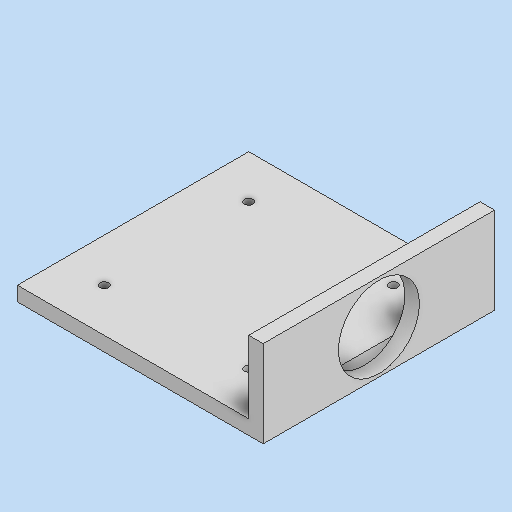
# Autodesk Inventor part: 电机底座
Saved by Autodesk Inventor 2026.2 (Build 302298010, 298A)
## iProperties
Created: 2026-03-16
Part Number: 电机底座
Material: 常规
Document SubType Name: Modeling
Designer: liu
Density: 1 g/cm^3
Appearance: 默认
Author: liu
Autodesk Inventor part; units mm, degrees
ref_plane "YZ Plane" through (0, 0, 0) normal (1, 0, 0) x (0, 1, 0)
ref_plane "XZ Plane" through (0, 0, 0) normal (0, 1, 0) x (-1, 0, 0)
ref_plane "XY Plane" through (0, 0, 0) normal (0, 0, 1) x (1, 0, 0)
sketch "草图1" plane through (0, 0, 0) normal (0, 1, 0) x (-1, 0, 0)
  line L0 (18.0685, 16.7445) -> (-61.9315, 16.7445)
  line L1 (-61.9315, 16.7445) -> (-61.9315, -63.2555)
  line L2 (-61.9315, -63.2555) -> (18.0685, -63.2555)
  line L3 (18.0685, -63.2555) -> (18.0685, 16.7445)
  point P0 (0, 0)
  dimension "d0" = 80
  dimension "d1" = 80
  constraints: 8 end point, 2 parallel, 1 horizontal, 1 perpendicular
  measures "d0" distance of L2.end L0.start
  measures "d1" distance of L0.start L0.end
extrude "拉伸1" add sketch "草图1" along normal blind 5
sketch "草图2" plane through (0, 5, 0) normal (0, 1, 0) x (1, 0, 0)
  circle A0 centre (46.9315, -1.7445) radius 1.5
  line L0 (61.9315, -16.7445) -> (61.9315, 63.2555) projected
  line L1 (-18.0685, -16.7445) -> (61.9315, -16.7445) projected
  circle A1 centre (-3.0685, -1.7445) radius 1.5
  circle A2 centre (-3.0685, 48.2555) radius 1.5
  circle A3 centre (46.9315, 48.2555) radius 1.5
  point P0 (0, 0)
  dimension "d4" = 15
  dimension "d5" = 15
  dimension "d6" = 3
  dimension "d9" = 50
  dimension "d16" = 50
  dimension "d23" = 50
  constraints: 4 centre point, 2 vertical, 1 horizontal, 6 other
  measures "d4" distance from line of L0 A0.centre
  measures "d5" distance from line of L1 A0.centre
  measures "d6" diameter of A0
  measures "d9" distance of A0.centre A1.centre
  measures "d16" distance of A1.centre A2.centre
  measures "d23" distance of A0.centre A3.centre
extrude "拉伸2" cut sketch "草图2" against normal blind 5
sketch "草图3" plane through (61.9315, 0, 16.7445) normal (1, 0, 0) x (0, 0, -1)
  line L0 (0, 30) -> (80, 30)
  line L1 (80, 30) -> (80, 0)
  line L2 (80, 0) -> (0, 0)
  line L3 (0, 0) -> (0, 30)
  line L4 (0, 0) -> (80, 0) projected
  line L5 (0, 0) -> (0, 5) projected
  point P0 (16.7445, 0)
  point P1 (0, 2.5)
  point P2 (0, 15)
  dimension "d30" = 30
  dimension "d31" = 80
  dimension "d32" = 0
  dimension "d33" = 0
  constraints: 8 end point, 2 midpoint, 2 parallel, 1 horizontal, 1 perpendicular
  measures "d30" distance of L2.end L0.start
  measures "d31" distance of L0.start L0.end
  measures "d32" distance between parallel lines of L4 L2
  measures "d33" horizontal distance of point (0, 2.5) point (0, 15)
extrude "拉伸3" add sketch "草图3" along normal blind 5
sketch "草图4" plane through (66.9315, 0, 16.7445) normal (1, 0, 0) x (0, 0, -1)
  circle A0 centre (40, 15) radius 14
  line L0 (0, 30) -> (0, 0) projected
  line L1 (0, 0) -> (80, 0) projected
  point P0 (16.7445, 0)
  point P1 (40, 0)
  dimension "d36" = 28
  dimension "d37" = 40
  dimension "d38" = 15
  constraints: 1 centre point, 1 midpoint
  measures "d36" diameter of A0
  measures "d37" distance from line of L0 A0.centre
  measures "d38" distance of point (40, 0) A0.centre
extrude "拉伸4" cut sketch "草图4" against normal blind 5
